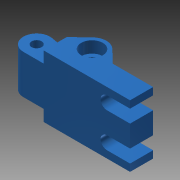
# Autodesk Inventor part: Infill3DIdler
Saved by Autodesk Inventor 2015 SP1 (Build 190203100, 203)
## iProperties
Created: 2015-04-27
Part Number: Infill3DIdler
Material: Generic
Document SubType Name: Modeling
Designer: Jack
Density: 1 g/cm^3
Appearance: Cyan
Author: Jack
Autodesk Inventor part; units mm, degrees
ref_plane "YZ Plane" through (0, 0, 0) normal (1, 0, 0) x (0, 1, 0)
ref_plane "XZ Plane" through (0, 0, 0) normal (0, 1, 0) x (-1, 0, 0)
ref_plane "XY Plane" through (0, 0, 0) normal (0, 0, 1) x (1, 0, 0)
sketch "Sketch1" plane through (0, 0, 0) normal (0, 0, 1) x (1, 0, 0)
  line L0 (0, 0) -> (30, 0)
  line L1 (30, 0) -> (30, 8)
  arc A0 (11.4837, 12.3867) -> (4.5163, 12.3867) centre (8, 8.8) ccw
  line L2 (30, 8) -> (16, 8)
  line L3 (0, 0) -> (0, 8)
  line L4 (0, 8) -> (4.5163, 12.3867)
  line L5 (11.4837, 12.3867) -> (16, 8)
  dimension "d0" = 8
  dimension "d1" = 30
  dimension "d2" = 22
  dimension "d3" = 8.8
  dimension "d4" = 10
  dimension "d5" = 8
  constraints: 12 end point, 2 horizontal, 2 point on circle, 2 tangent, 1 centre point, 1 equal length, 1 perpendicular, 1 vertical
  measures "d0" distance of L0.end L1.end
  measures "d1" distance of L0.start L0.end
  measures "d2" horizontal distance of L1.end A0.centre
  measures "d3" distance from line of L0 A0.centre
  measures "d4" diameter of A0
  measures "d5" distance of L0.start L3.end
extrude "Extrusion1" add sketch "Sketch1" along normal blind 21.5
ref_plane "Work Plane1" through (0, 0, 10.75) normal (0, 0, 1) x (1, 0, 0)
sketch "Sketch2" plane through (0, 0, 10.75) normal (0, 0, 1) x (1, 0, 0)
  arc A0 (11.4837, 12.3867) -> (4.5163, 12.3867) centre (8, 8.8) ccw projected
  arc A1 (-6.1752, 9.1255) -> (-7, 0) centre (-7, 4.6) ccw
  line L0 (-6.1752, 9.1255) -> (0, 8)
  line L1 (-7, 0) -> (0, 0)
  line L2 (0, 8) -> (0, 0)
  dimension "d10" = 15
  dimension "d11" = 9.2
  constraints: 6 end point, 2 point on circle, 2 tangent, 1 centre point, 1 horizontal, 1 vertical
  measures "d10" horizontal distance of A1.centre A0.centre
  measures "d11" diameter of A1
extrude "Extrusion2" add sketch "Sketch2" along normal mid plane 13.6
sketch "Sketch3" plane through (0, 0, 17.55) normal (0, 0, 1) x (1, 0, 0)
  arc A0 (-6.1752, 9.1255) -> (-7, 0) centre (-7, 4.6) ccw projected
hole "Hole1" at (-7, 4.6, 17.55) direction (0, 0, -1) diameter 3.5 end through all
sketch "Sketch4" plane through (0, 0, 21.5) normal (0, 0, 1) x (1, 0, 0)
  arc A0 (11.4837, 12.3867) -> (4.5163, 12.3867) centre (8, 8.8) ccw projected
hole "Hole2" at (8, 8.8, 21.5) direction (0, 0, -1) diameter 4.5 end through all
ref_plane "Work Plane2" through (0, 0, 11.5) normal (0, 0, 1) x (1, 0, 0)
sketch "Sketch5" plane through (0, 0, 11.5) normal (0, 0, 1) x (1, 0, 0)
  circle A0 centre (8, 8.8) radius 2.25 projected
  circle A1 centre (8, 8.8) radius 8
  point P0 (0, 0)
  dimension "d29" = 16
  constraints: 1 centre point, 1 coincident
  measures "d29" diameter of A1
extrude "Extrusion3" cut sketch "Sketch5" along normal mid plane 7
sketch "Sketch6" plane through (0, 0, 21.5) normal (0, 0, 1) x (1, 0, 0)
  circle A0 centre (8, 8.8) radius 2.25 projected
hole "Hole3" at (8, 8.8, 21.5) direction (0, 0, -1) diameter 7.5 depth 4
sketch "Sketch7" plane through (0, 0, 0) normal (0, 0, -1) x (-1, 0, 0)
  circle A0 centre (-8, 8.8) radius 2.25 projected
  arc A1 (-4.5163, 12.3867) -> (-11.4837, 12.3867) centre (-8, 8.8) ccw projected
  line L0 (-8, 4.5276) -> (-11.7, 6.6638)
  line L1 (-11.7, 6.6638) -> (-11.7, 10.9362)
  line L2 (-11.7, 10.9362) -> (-8, 13.0724)
  line L3 (-8, 13.0724) -> (-4.3, 10.9362)
  line L4 (-4.3, 10.9362) -> (-4.3, 6.6638)
  line L5 (-4.3, 6.6638) -> (-8, 4.5276)
  dimension "d39" = 7.4
  constraints: 12 end point, 1 coincident, 1 vertical, 13 other
  measures "d39" distance between parallel lines of L4 L1
extrude "Extrusion4" cut sketch "Sketch7" against normal blind 3.5
sketch "Sketch8" plane through (0, 0, 8) normal (0, 0, 1) x (1, 0, 0)
  circle A0 centre (8, 8.8) radius 2.25 projected
  circle A1 centre (8, 8.8) radius 5
  point P0 (0, 0)
  dimension "d42" = 10
  constraints: 1 centre point, 1 coincident
  measures "d42" diameter of A1
extrude "Extrusion5" add sketch "Sketch8" along normal blind 1
sketch "Sketch9" plane through (0, 0, 15) normal (0, 0, -1) x (-1, 0, 0)
  arc A0 (-4.5163, 12.3867) -> (-11.4837, 12.3867) centre (-8, 8.8) ccw projected
  circle A1 centre (-8, 8.8) radius 2.25 projected
  circle A2 centre (-8, 8.8) radius 5
  point P0 (0, 0)
  constraints: 1 centre point, 1 coincident, 1 concentric
extrude "Extrusion6" add sketch "Sketch9" along normal blind 1
chamfer "Chamfer1" distance 1 angle 45 2 edges at (3, 8.8, 9) (13, 8.8, 14)
sketch "Sketch10" plane through (0, 0, 0) normal (0, -1, 0) x (1, 0, 0)
  line L0 (30, 0) -> (30, 21.5) projected
  line L1 (0, 21.5) -> (30, 21.5) projected
  arc A0 (22, 19) -> (22, 14.5) centre (22, 16.75) ccw
  arc A1 (22, 7) -> (22, 2.5) centre (22, 4.75) ccw
  line L2 (22, 2.5) -> (30, 2.5)
  line L3 (22, 7) -> (30, 7)
  line L4 (22, 14.5) -> (30, 14.5)
  line L5 (22, 19) -> (30, 19)
  dimension "d50" = 4.5
  dimension "d51" = 12
  dimension "d52" = 4.75
  dimension "d53" = 8
  constraints: 8 end point, 4 perpendicular, 4 point on circle, 4 point on line, 4 tangent, 2 centre point, 1 equal radius, 1 vertical alignment
  measures "d50" diameter of A1
  measures "d51" distance of A0.centre A1.centre
  measures "d52" distance from line of L1 A0.centre
  measures "d53" distance from line of L0 A0.centre
extrude "Extrusion7" cut sketch "Sketch10" against normal up to next
body "Solid1"
